Autodesk Inventor part; units mm, degrees
(part 2 of 2)
sketch "Pattern_2_SKETCH_36" plane through (45.72, 0, 0) normal (0, 1, 0) x (1, 0, 0)
  line L0 (0.381, 0.508) -> (0.381, -0.508)
  line L1 (0.381, -0.508) -> (0.762, -0.508)
  line L2 (0.762, -0.508) -> (0.762, 0.508)
  line L3 (0.762, 0.508) -> (0.381, 0.508)
  constraints: 8 end point
sketch "Pattern_2_SKETCH_37" plane through (47.3456, 0, 0) normal (0, 1, 0) x (1, 0, 0)
  line L0 (0.381, 0.508) -> (0.381, -0.508)
  line L1 (0.381, -0.508) -> (0.762, -0.508)
  line L2 (0.762, -0.508) -> (0.762, 0.508)
  line L3 (0.762, 0.508) -> (0.381, 0.508)
  constraints: 8 end point
sketch "Pattern_2_SKETCH_38" plane through (48.26, 0, 0) normal (0, 1, 0) x (1, 0, 0)
  line L0 (0.381, 0.508) -> (0.381, -0.508)
  line L1 (0.381, -0.508) -> (0.762, -0.508)
  line L2 (0.762, -0.508) -> (0.762, 0.508)
  line L3 (0.762, 0.508) -> (0.381, 0.508)
  constraints: 8 end point
sketch "Pattern_2_SKETCH_39" plane through (49.8856, 0, 0) normal (0, 1, 0) x (1, 0, 0)
  line L0 (0.381, 0.508) -> (0.381, -0.508)
  line L1 (0.381, -0.508) -> (0.762, -0.508)
  line L2 (0.762, -0.508) -> (0.762, 0.508)
  line L3 (0.762, 0.508) -> (0.381, 0.508)
  constraints: 8 end point
extrude "Extrusion83" add sketch "Pattern_2_SKETCH_1" along normal blind 7.366
extrude "Extrusion84" add sketch "Pattern_2_SKETCH_2" along normal blind 7.366
extrude "Extrusion85" add sketch "Pattern_2_SKETCH_3" along normal blind 7.366
extrude "Extrusion86" add sketch "Pattern_2_SKETCH_4" along normal blind 7.366
extrude "Extrusion87" add sketch "Pattern_2_SKETCH_5" along normal blind 7.366
extrude "Extrusion88" add sketch "Pattern_2_SKETCH_6" along normal blind 7.366
extrude "Extrusion89" add sketch "Pattern_2_SKETCH_7" along normal blind 7.366
extrude "Extrusion90" add sketch "Pattern_2_SKETCH_8" along normal blind 7.366
extrude "Extrusion91" add sketch "Pattern_2_SKETCH_9" along normal blind 7.366
extrude "Extrusion92" add sketch "Pattern_2_SKETCH_10" along normal blind 7.366
extrude "Extrusion93" add sketch "Pattern_2_SKETCH_11" along normal blind 7.366
extrude "Extrusion94" add sketch "Pattern_2_SKETCH_12" along normal blind 7.366
extrude "Extrusion95" add sketch "Pattern_2_SKETCH_13" along normal blind 7.366
extrude "Extrusion96" add sketch "Pattern_2_SKETCH_14" along normal blind 7.366
extrude "Extrusion97" add sketch "Pattern_2_SKETCH_15" along normal blind 7.366
extrude "Extrusion98" add sketch "Pattern_2_SKETCH_16" along normal blind 7.366
extrude "Extrusion99" add sketch "Pattern_2_SKETCH_17" along normal blind 7.366
extrude "Extrusion100" add sketch "Pattern_2_SKETCH_18" along normal blind 7.366
extrude "Extrusion101" add sketch "Pattern_2_SKETCH_19" along normal blind 7.366
extrude "Extrusion102" add sketch "Pattern_2_SKETCH_20" along normal blind 7.366
extrude "Extrusion103" add sketch "Pattern_2_SKETCH_21" along normal blind 7.366
extrude "Extrusion104" add sketch "Pattern_2_SKETCH_22" along normal blind 7.366
extrude "Extrusion105" add sketch "Pattern_2_SKETCH_23" along normal blind 7.366
extrude "Extrusion106" add sketch "Pattern_2_SKETCH_24" along normal blind 7.366
extrude "Extrusion107" add sketch "Pattern_2_SKETCH_25" along normal blind 7.366
extrude "Extrusion108" add sketch "Pattern_2_SKETCH_26" along normal blind 7.366
extrude "Extrusion109" add sketch "Pattern_2_SKETCH_27" along normal blind 7.366
extrude "Extrusion110" add sketch "Pattern_2_SKETCH_28" along normal blind 7.366
extrude "Extrusion111" add sketch "Pattern_2_SKETCH_29" along normal blind 7.366
extrude "Extrusion112" add sketch "Pattern_2_SKETCH_30" along normal blind 7.366
extrude "Extrusion113" add sketch "Pattern_2_SKETCH_31" along normal blind 7.366
extrude "Extrusion114" add sketch "Pattern_2_SKETCH_32" along normal blind 7.366
extrude "Extrusion115" add sketch "Pattern_2_SKETCH_33" along normal blind 7.366
extrude "Extrusion116" add sketch "Pattern_2_SKETCH_34" along normal blind 7.366
extrude "Extrusion117" add sketch "Pattern_2_SKETCH_35" along normal blind 7.366
extrude "Extrusion118" add sketch "Pattern_2_SKETCH_36" along normal blind 7.366
extrude "Extrusion119" add sketch "Pattern_2_SKETCH_37" along normal blind 7.366
extrude "Extrusion120" add sketch "Pattern_2_SKETCH_38" along normal blind 7.366
extrude "Extrusion121" add sketch "Pattern_2_SKETCH_39" along normal blind 7.366
ref_plane "bottom_socket_XY" through (25.527, 0, 0) normal (0, 1, 0) x (1, 0, 0)
ref_plane "bottom_socket_YZ" through (25.527, 0, 0) normal (1, 0, 0) x (0, 0, -1)
ref_plane "bottom_socket_ZX" through (25.527, 0, 0) normal (0, 0, -1) x (0, 1, 0)
body "Solid1"
